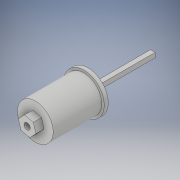
# Autodesk Inventor part: drive shaft
Saved by Autodesk Inventor 2018 (Build 220112000, 112)
## iProperties
Created: 2018-01-27
Part Number: drive shaft
Material: Generic
Document SubType Name: Modeling
Designer: prakh
Density: 1 g/cm^3
Appearance: Default
Author: prakh
Autodesk Inventor part; units mm, degrees
ref_plane "YZ Plane" through (0, 0, 0) normal (1, 0, 0) x (0, 1, 0)
ref_plane "XZ Plane" through (0, 0, 0) normal (0, 1, 0) x (-1, 0, 0)
ref_plane "XY Plane" through (0, 0, 0) normal (0, 0, 1) x (1, 0, 0)
sketch "Sketch1" plane through (0, 0, 0) normal (0, 0, 1) x (1, 0, 0)
  circle A0 centre (0, 0) radius 15.875
  dimension "d0" = 31.75
  constraints: 1 centre point, 1 coincident
  measures "d0" diameter of A0
extrude "Extrusion1" add sketch "Sketch1" along normal blind 3.175
sketch "Sketch2" plane through (0, 0, 3.175) normal (0, 0, 1) x (1, 0, 0)
  circle A0 centre (0, 0) radius 14.0335
  dimension "d3" = 28.067
  constraints: 1 centre point, 1 coincident
  measures "d3" diameter of A0
extrude "Extrusion2" add sketch "Sketch2" along normal blind 38.1
sketch "Sketch3" plane through (0, 0, 41.275) normal (0, 0, 1) x (1, 0, 0)
  line L0 (6.851, -1.6161) -> (2.0259, -6.7412)
  line L1 (2.0259, -6.7412) -> (-4.8251, -5.1251)
  line L2 (-4.8251, -5.1251) -> (-6.851, 1.6161)
  line L3 (-6.851, 1.6161) -> (-2.0259, 6.7412)
  line L4 (-2.0259, 6.7412) -> (4.8251, 5.1251)
  line L5 (4.8251, 5.1251) -> (6.851, -1.6161)
  point P0 (0, 0)
  point P1 (0, 0)
  dimension "d6" = 12.192
  constraints: 12 end point, 1 coincident, 13 other
  measures "d6" distance between parallel lines of L3 L0
extrude "Extrusion3" add sketch "Sketch3" along normal blind 6.35
sketch "Sketch4" plane through (0, 0, 47.625) normal (0, 0, 1) x (1, 0, 0)
  circle A0 centre (0, 0) radius 2.4511
  dimension "d9" = 4.9022
  constraints: 1 centre point, 1 coincident
  measures "d9" diameter of A0
extrude "Extrusion4" cut sketch "Sketch4" against normal blind 19.05
sketch "Sketch5" plane through (0, 0, 0) normal (0, 0, -1) x (-1, 0, 0)
  line L0 (1.8415, 1.8415) -> (-1.8415, 1.8415)
  line L1 (-1.8415, 1.8415) -> (-1.8415, -1.8415)
  line L2 (-1.8415, -1.8415) -> (1.8415, -1.8415)
  line L3 (1.8415, -1.8415) -> (1.8415, 1.8415)
  point P0 (0, 0)
  point P1 (0, -1.8415)
  point P2 (1.8415, 0)
  dimension "d12" = 3.683
  constraints: 8 end point, 2 midpoint, 2 parallel, 2 perpendicular, 1 horizontal, 1 horizontal alignment, 1 vertical alignment
  measures "d12" distance between parallel lines of L2 L0
extrude "Extrusion5" add sketch "Sketch5" along normal blind 50.8
sketch "Sketch6" plane through (0, 0, 0) normal (0, 0, -1) x (-1, 0, 0)
  point P0 (0, 0)
body "Solid1"
